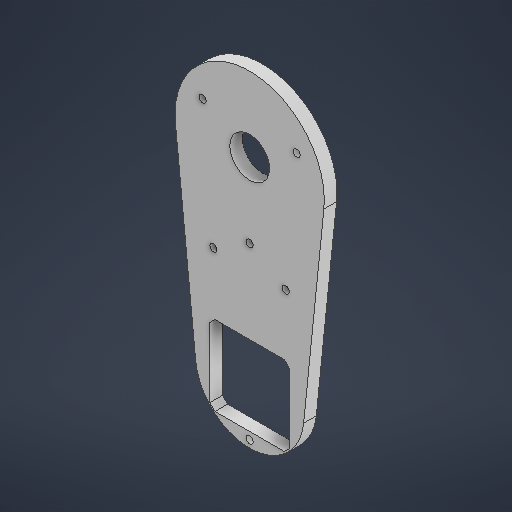
# Autodesk Inventor part: SupNema1
Saved by Autodesk Inventor 2025.3 (Build 293356000, 356)
## iProperties
Created: 2025-04-19
Part Number: SupNema1
Material: Generic
Document SubType Name: Modeling
Designer: Nelson
Density: 1 g/cm^3
Appearance: Default
Author: Nelson
Autodesk Inventor part; units mm, degrees
ref_plane "YZ Plane" through (0, 0, 0) normal (1, 0, 0) x (0, 1, 0)
ref_plane "XZ Plane" through (0, 0, 0) normal (0, 1, 0) x (-1, 0, 0)
ref_plane "XY Plane" through (0, 0, 0) normal (0, 0, 1) x (1, 0, 0)
ref_plane "Work Plane1" through (0, 0, 0) normal (0, 0, 1) x (1, 0, 0)
sketch "Sketch1" plane through (0, 0, 0) normal (0, 0, 1) x (1, 0, 0)
  line L0 (0, 0) -> (0, 53.385) construction
  line L1 (0, 0) -> (0, -55.885)
  circle A0 centre (0, 53.385) radius 11
  line L2 (22, -77.885) -> (-22, -33.885) construction
  line L3 (-22, -77.885) -> (22, -33.885) construction
  circle A1 centre (0, -55.885) radius 30
  circle A2 centre (0, 53.385) radius 41.25
  line L4 (-29.8406, -58.9737) -> (-41.0308, 49.1381)
  line L5 (29.8406, -58.9737) -> (41.0308, 49.1381)
  line L6 (22, -77.885) -> (20.5858, -76.4708)
  line L7 (20.5858, -76.4708) -> (22, -75.0566)
  line L8 (20.5858, -76.4708) -> (19.1716, -77.885)
  line L9 (20.5858, -35.2992) -> (19.1716, -33.885)
  line L10 (20.5858, -35.2992) -> (22, -36.7134)
  line L11 (-20.5858, -35.2992) -> (-22, -36.7134)
  line L12 (-20.5858, -35.2992) -> (-19.1716, -33.885)
  line L13 (-20.5858, -76.4708) -> (-19.1716, -77.885)
  line L14 (-20.5858, -76.4708) -> (-22, -75.0566)
  line L15 (22, -76.2811) -> (22, -77.885)
  line L16 (22, -77.885) -> (20.3961, -77.885)
  line L17 (22, -33.885) -> (22, -35.4889)
  line L18 (22, -36.7134) -> (22, -75.0566)
  line L19 (20.3961, -33.885) -> (22, -33.885)
  line L20 (-22, -33.885) -> (-20.3961, -33.885)
  line L21 (-19.1716, -33.885) -> (19.1716, -33.885)
  line L22 (-22, -35.4889) -> (-22, -33.885)
  line L23 (-22, -77.885) -> (-22, -76.2811)
  line L24 (-22, -75.0566) -> (-22, -36.7134)
  line L25 (19.1716, -77.885) -> (-19.1716, -77.885)
  line L26 (-20.3961, -77.885) -> (-22, -77.885)
  line L27 (22, -35.4889) -> (22, -36.7134)
  line L28 (20.3961, -33.885) -> (19.1716, -33.885)
  line L29 (-20.3961, -33.885) -> (-19.1716, -33.885)
  line L30 (-22, -35.4889) -> (-22, -36.7134)
  line L31 (-22, -76.2811) -> (-22, -75.0566)
  line L32 (-20.3961, -77.885) -> (-19.1716, -77.885)
  line L33 (19.1716, -77.885) -> (20.3961, -77.885)
  line L34 (22, -76.2811) -> (22, -75.0566)
  circle A3 centre (0, 53.385) radius 30
  circle A4 centre (0, 23.385) radius 2 construction
  circle A5 centre (25.9808, 68.385) radius 2
  circle A6 centre (-25.9808, 68.385) radius 2
  circle A7 centre (0, 83.385) radius 5
  line L35 (-16, 83.385) -> (16, 83.385) construction
  circle A8 centre (16, 83.385) radius 1.75
  circle A9 centre (-16, 83.385) radius 1.75
  circle A10 centre (-17.9808, 24.5286) radius 1.75
  circle A11 centre (-25.9808, 38.385) radius 5
  circle A12 centre (-33.9808, 52.2414) radius 1.75
  circle A13 centre (33.9808, 52.2414) radius 1.75
  circle A14 centre (25.9808, 38.385) radius 5
  circle A15 centre (17.9808, 24.5286) radius 1.75
  line L36 (0, -85.885) -> (0, -81.885)
  circle A16 centre (0, -81.885) radius 2
  line L37 (0, 0) -> (-20, 0)
  line L38 (0, 0) -> (20, 0)
  circle A17 centre (20, 0) radius 2
  circle A18 centre (-20, 0) radius 2
  circle A19 centre (-25.9808, 38.385) radius 11 construction
  circle A20 centre (25.9808, 38.385) radius 11 construction
  circle A21 centre (0, 83.385) radius 11 construction
  circle A22 centre (0, 12.135) radius 2
  line L39 (0, 53.385) -> (0, 31.385)
  circle A23 centre (0, 31.385) radius 4.5
  dimension "d5" = 60
  dimension "d0" = 53.385
  dimension "d1" = 55.885
  dimension "d2" = 22
  dimension "d3" = 44
  dimension "d4" = 44
  dimension "d6" = 82.5
  dimension "d7" = 2
  dimension "d10" = 360
  dimension "d14" = 60
  dimension "d15" = 4
  dimension "d18" = 360
  dimension "d22" = 10
  dimension "d29" = 32
  dimension "d30" = 3.5
  dimension "Fu" = 3.5
  dimension "d34" = 360
  dimension "d38" = 4
  dimension "d39" = 4
  dimension "d40" = 20
  dimension "d41" = 20
  dimension "d42" = 4
  dimension "d43" = 22
  dimension "d46" = 360
  dimension "d48" = 4
  dimension "Lean" = 9
  dimension "d50" = 22
  constraints: 80 end point, 23 centre point, 18 parallel, 13 perpendicular, 11 coincident, 8 point on line, 5 collinear, 5 horizontal, 5 point on circle, 3 midpoint, 3 tangent, 2 vertical, 69 other
  measures "d0" distance of L0.start L0.end
  measures "d1" distance of L0.start L1.end
  measures "d2" diameter of A0
  measures "d3" distance of L2.end L3.end
  measures "d4" distance of L3.start L2.end
  measures "d6" diameter of A2
  measures "d7" distance of L2.start L6.end
  measures "d14" diameter of A3
  measures "d15" diameter of A4
  measures "d22" diameter of A7
  measures "d29" distance of L35.start L35.end
  measures "d30" diameter of A8
  measures "Fu" diameter of A9
  measures "d38" distance of L36.start L36.end
  measures "d39" diameter of A16
  measures "d40" distance of L0.start L37.end
  measures "d41" distance of L0.start L38.end
  measures "d42" diameter of A18
  measures "d43" diameter of A19
  measures "d48" diameter of A22
  measures "Lean" diameter of A23
  measures "d50" distance of L39.start L39.end
extrude "Extrusion1" add sketch "Sketch1" along normal blind 7 contours A1 L28 L21 L1 | A1 L20 L22 L4 A2 A22 L5 L17 L19 | L1 L21 L29 A1 | L19 L17 A1 | A1 L27 L10 L9 L28 | L29 L12 L11 L30 A1 | A1 L22 L20 | A1 L34 L18 L27 | L30 L24 L31 A1 | L34 A1 L6 L7 | L31 L14 L13 L32 A1 | A2 A22 | L6 A1 L33 L8 | L32 L25 L33 A1 | A22 A2 | A2 A22 | A3 A14 A11 A6 A7 A5 | A5 A3 | A3 A5 | A14 A3 | A3 A14 | A7 A3 | A3 A7 | A11 A3 | A3 A11 | A6 A3 | A3 A6 | A8 | A9 | A10 | A12 | A13 | A15 | A16 | A17 | A18 | A23
extrude "Extrusion2" cut sketch "Sketch1" along normal up to surface (7 mm away) contours A22 A2 | A2 A22 | A5 A3 | A3 A5 | A6 A3 | A3 A6 | A16 | A17 | A18 picked at (-0.0791, 12.8005) picked at (0.0729, 11.4759)
extrude "Extrusion3" cut sketch "Sketch1" along normal blind 5 contours A14 A3 | A3 A14 | A7 A3 | A3 A7 | A11 A3 | A3 A11 | A23
extrude "Extrusion4" cut sketch "Sketch1" along normal blind 3 contours A8 | A9 | A10 | A12 | A13 | A15
equation "\"d30\" = Fu"
body "Solid1"
